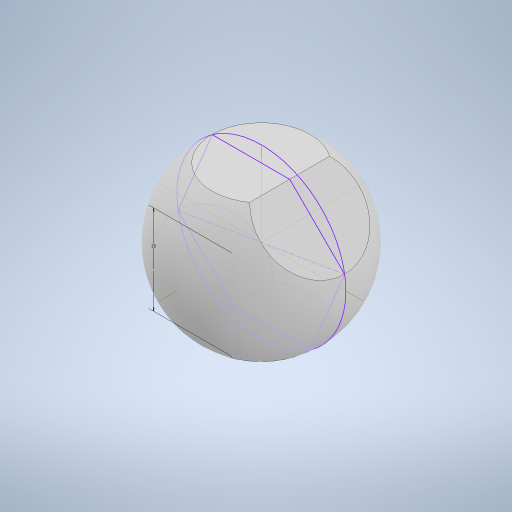
# Autodesk Inventor part: D20-2
Saved by Autodesk Inventor 2023 (Build 270158030, 158C)
## iProperties
Created: 2024-08-24
Part Number: D20-2
Material: Generic
Document SubType Name: Modeling
Designer: Imogen Heard
Density: 1 g/cm^3
Appearance: Default
Author: Imogen Heard
Autodesk Inventor part; units mm, degrees
ref_plane "YZ Plane" through (0, 0, 0) normal (1, 0, 0) x (0, 1, 0)
ref_plane "XZ Plane" through (0, 0, 0) normal (0, 1, 0) x (-1, 0, 0)
ref_plane "XY Plane" through (0, 0, 0) normal (0, 0, 1) x (1, 0, 0)
sketch "Sketch12" plane through (0, 0, 0) normal (0, 0, 1) x (1, 0, 0)
  line L0 (10.9683, -15.3581) -> (-6.3522, -25.3581) construction
  line L1 (-6.3522, -25.3581) -> (-6.3522, -5.3581) construction
  line L2 (-6.3522, -5.3581) -> (10.9683, -15.3581) construction
  circle A0 centre (0, 0) radius 18.8726
  line L3 (-18.6124, -3.1234) -> (-10.9683, 15.3581)
  line L4 (-10.9683, 15.3581) -> (6.3522, 15.3581)
  line L5 (6.3522, 15.3581) -> (18.6124, 3.1234)
  line L6 (10.9683, -15.3581) -> (18.6124, 3.1234)
  line L7 (10.9683, -15.3581) -> (-6.3522, -15.3581)
  line L8 (-6.3522, -15.3581) -> (-18.6124, -3.1234)
  line L9 (-18.6124, -3.1234) -> (18.6124, 3.1234)
  dimension "d49" = 20
  dimension "d36" = 20
  constraints: 20 end point, 6 equal length, 4 point on circle, 3 midpoint, 2 coincident, 2 horizontal, 1 centre point, 1 vertical
  measures "d49" distance of L0.end L1.end
revolve "Revolution2" add sketch "Sketch12" angle 360 about axis through (-18.6124, -3.1234, 0) along (0.9862099, 0.1654995, 0) contours L5 L4 A0 | L9 L3 L4 L5 | L3 A0
extrude "Extrusion6" cut sketch "Sketch12" along normal through all both and the other way through all contours L5 L4 A0 | A0 L8 L7
body "Solid4"
body "Solid5"
